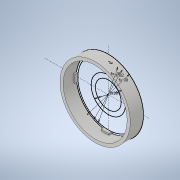
# Autodesk Inventor part: hall_case
Saved by Autodesk Inventor 2020 (Build 240168000, 168)
## iProperties
Created: 2018-05-11
Part Number: hall_case
Material: Generic
Document SubType Name: Modeling
Designer: stedrock
Density: 1 g/cm^3
Appearance: Default
Mass: 28.3178 g
Surface Area: 160.353 cm^2
Volume: 28.3178 cm^3
Author: stedrock
Autodesk Inventor part; units mm, degrees
ref_plane "YZ Plane" through (0, 0, 0) normal (1, 0, 0) x (0, 1, 0)
ref_plane "XZ Plane" through (0, 0, 0) normal (0, 1, 0) x (-1, 0, 0)
ref_plane "XY Plane" through (0, 0, 0) normal (0, 0, 1) x (1, 0, 0)
sketch "Sketch1" plane through (0, 0, 0) normal (0, 0, 1) x (1, 0, 0)
  circle A0 centre (0, 0) radius 16.5
  circle A1 centre (0, 0) radius 22
  circle A2 centre (0, 0) radius 41
  circle A3 centre (0, 0) radius 45
  line L0 (0, 0) -> (-82.1679, 0) construction
  line L1 (0, 0) -> (52.3587, 0) construction
  line L2 (0, 0) -> (0, 55.2671) construction
  line L3 (0, 0) -> (0, -51.5979) construction
  circle A4 centre (0, 0) radius 39
  line L4 (5, 40.694) -> (5, 38.6782)
  line L5 (-5, 40.694) -> (-5, 38.6782)
  arc A5 (5, 40.694) -> (-5, 40.694) centre (0, 0) ccw
  arc A6 (5, 38.6782) -> (-5, 38.6782) centre (0, 0) ccw
  dimension "d2" = 82
  dimension "d15" = 78
  dimension "d0" = 33
  dimension "d1" = 44
  dimension "d3" = 90
  dimension "d16" = 5
  constraints: 12 end point, 5 centre point, 5 coincident, 4 point on circle, 3 vertical, 2 horizontal, 2 symmetric about line, 6 other
  measures "d0" diameter of A0
  measures "d1" diameter of A1
  measures "d3" diameter of A3
  measures "d16" distance between parallel lines of L2 L4
extrude "outer" add sketch "Sketch1" along normal blind 16.7 contours A3
extrude "inner" [suppressed]
extrude "Extrusion4" add sketch "Sketch1" along normal blind 4 contours L4 A4 L5 A2 picked at (3.8902, 39.4454)
pattern_circular "Circular Pattern1" count 4 over 360 about axis through (0, 0, -10) along (0, 0, 1) of "Extrusion4"
equation "\"d15\" = PCB_OD"
equation "\"d0\" = skeleton_OD"
equation "\"d1\" = PCB_ID"
equation "\"d3\" = carbon_OD"
equation "\"PCB_OD\" = 78"
equation "\"PCB_ID\" = 44"
equation "\"skeleton_OD\" = 33"
equation "\"carbon_OD\" = 90"
body "Solid1"
